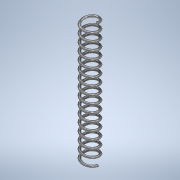
# Autodesk Inventor part: Peça 16
Saved by Autodesk Inventor 2021 (Build 250183000, 183)
## iProperties
Created: 2020-11-15
Part Number: Peça 16
Material: Liga de Nickel-Copper 400
Document SubType Name: Modeling
Designer: Bruno
Density: 8.83 g/cm^3
Appearance: Cromado - Preto polido
Author: Bruno
Autodesk Inventor part; units mm, degrees
ref_plane "YZ Plane" through (0, 0, 0) normal (1, 0, 0) x (0, 1, 0)
ref_plane "XZ Plane" through (0, 0, 0) normal (0, 1, 0) x (-1, 0, 0)
ref_plane "XY Plane" through (0, 0, 0) normal (0, 0, 1) x (1, 0, 0)
sketch "Esboço1" plane through (0, 0, 0) normal (0, 0, 1) x (1, 0, 0)
  circle A0 centre (0, 0) radius 1.25
  circle A1 centre (0, 0) radius 0.9
  circle A2 centre (1.075, 0) radius 0.175
  dimension "d0" = 1.8
  dimension "d1" = 2.5
  dimension "d2" = 0.35
  constraints: 3 centre point, 2 coincident, 1 tangent
  measures "d0" diameter of A1
  measures "d1" diameter of A0
  measures "d2" diameter of A2
coil "Espiral1" sketch "Esboço1" operation add axis through (0, -10, 0) along (0, 1, 0) pitch 1.125 turns 16 hand left contours A2
